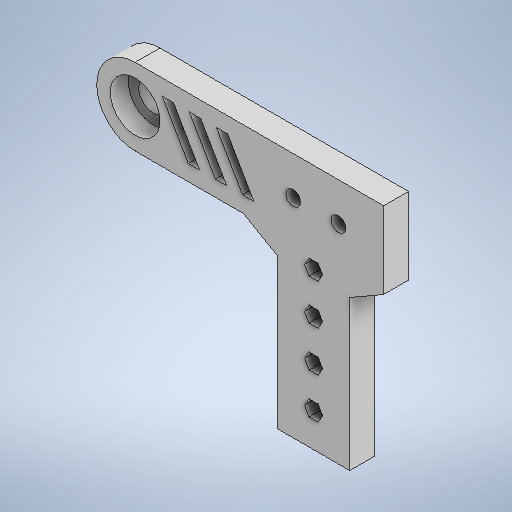
# Autodesk Inventor part: blet_leg_30x30 - rozsirene (zdcardlove)
Saved by Autodesk Inventor 2025 (Build 290162000, 162)
## iProperties
Created: 2024-12-16
Part Number: blet_leg_30x30 - rozsirene (zdcardlove)
Material: Všeobecné
Document SubType Name: Modeling
Designer: lukas
Density: 1 g/cm^3
Appearance: Výchozí
Author: lukas
## iProperties of the stored document blet_leg_30x30_3D tisk.ipt
Created: 2025-01-12
Part Number: blet_leg_30x30_3D tisk
Material: Všeobecné
Document SubType Name: Modeling
Designer: lukas
Density: 1 g/cm^3
Appearance: Výchozí
Author: lukas
Autodesk Inventor part; units mm, degrees
ref_plane "YZ Plane" through (0, 0, 0) normal (1, 0, 0) x (0, 1, 0)
ref_plane "XZ Plane" through (0, 0, 0) normal (0, 1, 0) x (-1, 0, 0)
ref_plane "XY Plane" through (0, 0, 0) normal (0, 0, 1) x (1, 0, 0)
sketch "Náčrt1" plane through (0, 0, 0) normal (0, 0, 1) x (1, 0, 0)
  line L0 (-97.4, 0) -> (80.4, 0) projected
  line L1 (0, -76.3) -> (0, 76.3) projected
  line L2 (-55, 54.5) -> (55, 54.5)
  line L3 (55, 54.5) -> (55, 20.5)
  line L4 (55, 20.5) -> (-55, 20.5)
  line L5 (-55, 20.5) -> (-55, 54.5)
  line L6 (40, -54.5) -> (8, -54.5)
  line L7 (8, -54.5) -> (8, 20.5)
  line L8 (8, 20.5) -> (40, 20.5)
  line L9 (40, 20.5) -> (40, -54.5)
  circle A0 centre (-55, 37.5) radius 17
  point P0 (0, 0)
  point P1 (-55, 20.5)
  dimension "d0" = 34
  dimension "d1" = 110
  dimension "d2" = 32
  dimension "d3" = 15
  dimension "d4" = 75
  constraints: 16 end point, 4 parallel, 2 horizontal, 2 perpendicular, 1 midpoint, 1 point on line, 5 other
  measures "d0" distance of L4.end L2.start
  measures "d1" distance of L2.start L2.end
  measures "d2" distance of L6.start L6.end
  measures "d3" distance from line of L3.end L9
  measures "d4" distance of L6.end L7.end
extrude "Vysunutí1" add sketch "Náčrt1" along normal blind 14 contours L7 L4 L9 L0 | L0 L9 L6 L7 | L4 A0 L2 L1 | L1 L2 L3 L4 | A0 L5 | L5 A0
sketch "Náčrt2" plane through (0, 0, 0) normal (0, 0, -1) x (-1, 0, 0)
  line L0 (-55, 54.5) -> (55, 54.5) projected
  line L1 (-55, 54.5) -> (55, 54.5) projected
  line L2 (-55, 20.5) -> (-55, 54.5) projected
  line L3 (-40, 20.5) -> (-55, 20.5) projected
  line L4 (-40, -54.5) -> (-40, 20.5) projected
  line L5 (-8, -54.5) -> (-40, -54.5) projected
  line L6 (-8, 20.5) -> (-8, -54.5) projected
  line L7 (55, 20.5) -> (-8, 20.5) projected
  arc A0 (55, 20.5) -> (55, 54.5) centre (55, 37.5) ccw projected
  point P0 (0, 0)
  constraints: 1 coincident
hole "Díra1" at (-55, 37.5, 0) direction (0, 0, 1) diameter 13 end through all counterbore diameter 22 counterbore depth 8
chamfer "Zkosení1" distance 3 angle 45 8 edges at (0, 54.5, 14) (-72, 37.5, 14) (-23.5, 20.5, 14) (8, -17, 14) (40, -17, 14) (47.5, 20.5, 14) (55, 37.5, 14) (24, -54.5, 14)
sketch "Náčrt3" plane through (0, 0, 14) normal (0, 0, 1) x (1, 0, 0)
  circle A0 centre (-55, 37.5) radius 6.5 projected
  line L0 (-55, 51.5) -> (52, 51.5) projected
  arc A1 (-55, 51.5) -> (-55, 23.5) centre (-55, 37.5) ccw projected
  line L1 (11, 23.5) -> (-55, 23.5) projected
  line L2 (11, -51.5) -> (11, 23.5) projected
  line L3 (37, -51.5) -> (11, -51.5) projected
  line L4 (37, 23.5) -> (37, -51.5) projected
  line L5 (52, 23.5) -> (37, 23.5) projected
  line L6 (52, 51.5) -> (52, 23.5) projected
  line L7 (0, 76.3) -> (0, -76.3) projected
  line L8 (-97.4, 0) -> (80.4, 0) projected
  point P0 (0, 0)
  point P1 (35, 37.5)
  dimension "d17" = 14
  dimension "d18" = 17
  measures "d17" distance from line of L0 point (35, 37.5)
  measures "d18" distance from line of L6 point (35, 37.5)
hole "Díra2" at (35, 37.5, 14) direction (0, 0, -1) diameter 6.5 end through all counterbore diameter 11 counterbore depth 4 clearance for "Strojní šroub se zápustnou hlavou" size "M6" standard "Ansi M metrický profil"
pattern_linear "Obdélníkové pole1" count 2 spacing 20 along (-1, 0, 0) of "Díra2"
sketch "Náčrt4" plane through (0, 0, 14) normal (0, 0, 1) x (1, 0, 0)
  line L0 (-97.4, 0) -> (80.4, 0) projected
  line L1 (0, -76.3) -> (0, 76.3) projected
  circle A0 centre (15, 37.5) radius 5.5 projected
  circle A1 centre (35, 37.5) radius 5.5 projected
  circle A2 centre (-55, 37.5) radius 6.5 projected
  line L2 (-55, 51.5) -> (52, 51.5) projected
  arc A3 (-55, 51.5) -> (-55, 23.5) centre (-55, 37.5) ccw projected
  line L3 (11, 23.5) -> (-55, 23.5) projected
  line L4 (11, -51.5) -> (11, 23.5) projected
  line L5 (37, -51.5) -> (11, -51.5) projected
  line L6 (37, 23.5) -> (37, -51.5) projected
  line L7 (52, 23.5) -> (37, 23.5) projected
  line L8 (52, 51.5) -> (52, 23.5) projected
  line L9 (-31.453, 27.5) -> (-26.453, 27.5)
  line L10 (-26.453, 27.5) -> (-38, 47.5)
  line L11 (-26.453, 27.5) -> (-3.359, 27.5) construction
  line L12 (-31.453, 27.5) -> (-43, 47.5)
  line L13 (-43, 47.5) -> (-38, 47.5)
  point P0 (0, 0)
  dimension "d29" = 120
  dimension "d31" = 5
  dimension "d32" = 4
  dimension "d33" = 4
  dimension "d34" = 12
  constraints: 10 end point, 3 horizontal, 1 equal length, 1 parallel
  measures "d29" angle of L11 L10
  measures "d31" distance of L12.end L10.end
  measures "d32" distance between parallel lines of L2 L13
  measures "d33" distance between parallel lines of L3 L9
  measures "d34" horizontal distance of A2.centre L12.end
extrude "Vysunutí2" cut sketch "Náčrt4" against normal through all contours L12 L13 L10 L9
chamfer "Zkosení2" distance 1 angle 45 4 edges at (-37.2265, 37.5, 14) (-40.5, 47.5, 14) (-32.2265, 37.5, 14) (-28.953, 27.5, 14)
pattern_linear "Obdélníkové pole2" count 3 spacing 12 along (1, 0, 0) of "Vysunutí2", "Zkosení2"
sketch "Náčrt5" plane through (0, 0, 14) normal (0, 0, 1) x (1, 0, 0)
  line L0 (-32.7321, 48.5) -> (-20.0303, 26.5) projected
  line L1 (-25.4226, 48.5) -> (-32.7321, 48.5) projected
  line L2 (-12.7209, 26.5) -> (-25.4226, 48.5) projected
  line L3 (-20.0303, 26.5) -> (-12.7209, 26.5) projected
  line L4 (-55, 51.5) -> (52, 51.5) projected
  arc A0 (-55, 51.5) -> (-55, 23.5) centre (-55, 37.5) ccw projected
  line L5 (11, 23.5) -> (-55, 23.5) projected
  line L6 (11, -51.5) -> (11, 23.5) projected
  line L7 (37, -51.5) -> (11, -51.5) projected
  line L8 (37, 23.5) -> (37, -51.5) projected
  line L9 (52, 23.5) -> (37, 23.5) projected
  line L10 (52, 51.5) -> (52, 23.5) projected
  circle A1 centre (-55, 37.5) radius 6.5 projected
  circle A2 centre (35, 37.5) radius 5.5 projected
  circle A3 centre (15, 37.5) radius 5.5 projected
  line L11 (-24.7209, 26.5) -> (-37.4226, 48.5) projected
  line L12 (-32.0303, 26.5) -> (-24.7209, 26.5) projected
  line L13 (-44.7321, 48.5) -> (-32.0303, 26.5) projected
  line L14 (-37.4226, 48.5) -> (-44.7321, 48.5) projected
  line L15 (-20.7321, 48.5) -> (-8.0303, 26.5) projected
  line L16 (-13.4226, 48.5) -> (-20.7321, 48.5) projected
  line L17 (-0.7209, 26.5) -> (-13.4226, 48.5) projected
  line L18 (-8.0303, 26.5) -> (-0.7209, 26.5) projected
  line L19 (0, -76.3) -> (0, 76.3) projected
  line L20 (26, 17.9641) -> (28, 14.5)
  line L21 (28, 14.5) -> (26, 11.0359)
  line L22 (26, 11.0359) -> (22, 11.0359)
  line L23 (22, 11.0359) -> (20, 14.5)
  line L24 (20, 14.5) -> (22, 17.9641)
  line L25 (22, 17.9641) -> (26, 17.9641)
  point P0 (0, 0)
  point P1 (24, 14.5)
  dimension "d43" = 4
  dimension "d44" = 9
  dimension "d45" = 13
  dimension "d52" = 3.4641
  constraints: 12 end point, 13 other
  measures "d43" distance of L24.end L20.start
  measures "d44" distance from line of L9 point (24, 14.5)
  measures "d45" distance from line of L8 point (24, 14.5)
  measures "d52" vertical distance of L23.end L24.end
extrude "Vysunutí3" cut sketch "Náčrt5" against normal through all contours L20 L21 L22 L23 L24 L25
chamfer "Zkosení3" distance 1 angle 45 6 edges at (24, 17.9641, 14) (27, 16.2321, 14) (27, 12.7679, 14) (24, 11.0359, 14) (21, 12.7679, 14) (21, 16.2321, 14)
pattern_linear "Obdélníkové pole3" count 4 spacing 18 along (0, -1, 0) of "Vysunutí3", "Zkosení3"
ref_plane "Pracovní rovina1" through (0, 0, 0) normal (0, 0, -1) x (-1, 0, 0)
sketch "Náčrt7" plane through (0, 0, 0) normal (0, 0, -1) x (-1, 0, 0)
  line L0 (-28, -39.5) -> (-26, -36.0359) projected
  line L1 (-26, -36.0359) -> (-22, -36.0359) projected
  line L2 (-22, -36.0359) -> (-20, -39.5) projected
  line L3 (-20, -39.5) -> (-22, -42.9641) projected
  line L4 (-22, -42.9641) -> (-26, -42.9641) projected
  line L5 (-26, -42.9641) -> (-28, -39.5) projected
  line L6 (-28, -21.5) -> (-26, -18.0359) projected
  line L7 (-26, -18.0359) -> (-22, -18.0359) projected
  line L8 (-22, -18.0359) -> (-20, -21.5) projected
  line L9 (-20, -21.5) -> (-22, -24.9641) projected
  line L10 (-22, -24.9641) -> (-26, -24.9641) projected
  line L11 (-26, -24.9641) -> (-28, -21.5) projected
  line L12 (-28, -3.5) -> (-26, -0.0359) projected
  line L13 (-26, -0.0359) -> (-22, -0.0359) projected
  line L14 (-22, -0.0359) -> (-20, -3.5) projected
  line L15 (-20, -3.5) -> (-22, -6.9641) projected
  line L16 (-22, -6.9641) -> (-26, -6.9641) projected
  line L17 (-26, -6.9641) -> (-28, -3.5) projected
  line L18 (-20, 14.5) -> (-22, 11.0359) projected
  line L19 (-22, 11.0359) -> (-26, 11.0359) projected
  line L20 (-26, 11.0359) -> (-28, 14.5) projected
  line L21 (-28, 14.5) -> (-26, 17.9641) projected
  line L22 (-26, 17.9641) -> (-22, 17.9641) projected
  line L23 (-22, 17.9641) -> (-20, 14.5) projected
  line L24 (19, 47.5) -> (7.453, 27.5) projected
  line L25 (7.453, 27.5) -> (2.453, 27.5) projected
  line L26 (2.453, 27.5) -> (14, 47.5) projected
  line L27 (14, 47.5) -> (19, 47.5) projected
  line L28 (31, 47.5) -> (19.453, 27.5) projected
  line L29 (19.453, 27.5) -> (14.453, 27.5) projected
  line L30 (14.453, 27.5) -> (26, 47.5) projected
  line L31 (26, 47.5) -> (31, 47.5) projected
  line L32 (26.453, 27.5) -> (38, 47.5) projected
  line L33 (38, 47.5) -> (43, 47.5) projected
  line L34 (43, 47.5) -> (31.453, 27.5) projected
  line L35 (31.453, 27.5) -> (26.453, 27.5) projected
  circle A0 centre (-15, 37.5) radius 3.25 projected
  circle A1 centre (-35, 37.5) radius 3.25 projected
  circle A2 centre (55, 37.5) radius 11 projected
  line L36 (-55, 54.5) -> (55, 54.5) projected
  line L37 (-55, 20.5) -> (-55, 54.5) projected
  line L38 (-40, 20.5) -> (-55, 20.5) projected
  line L39 (-40, -54.5) -> (-40, 20.5) projected
  line L40 (-8, -54.5) -> (-40, -54.5) projected
  line L41 (-8, 20.5) -> (-8, -54.5) projected
  line L42 (55, 20.5) -> (-8, 20.5) projected
  arc A3 (55, 20.5) -> (55, 54.5) centre (55, 37.5) ccw projected
  line L43 (-40, 11.8397) -> (-55, 20.5)
  line L44 (-8, 11.8397) -> (7, 20.5)
  line L45 (-8, 20.5) -> (-8, -54.5) projected
  line L46 (-8, 11.8397) -> (-8, 20.5)
  line L47 (-8, 20.5) -> (7, 20.5)
  line L48 (-40, -54.5) -> (-40, 20.5) projected
  line L49 (-40, 11.8397) -> (-40, 20.5)
  line L50 (-40, 20.5) -> (-55, 20.5)
  point P0 (0, 0)
  dimension "d68" = 15
  dimension "d69" = 15
  dimension "d70" = 30
  dimension "d71" = 30
  constraints: 12 end point, 4 collinear, 4 point on line
  measures "d68" distance of L38.start L43.end
  measures "d69" distance of L41.start L44.end
  measures "d70" angle of L42 L44
  measures "d71" angle of L38 L43
extrude "Vysunutí4" add sketch "Náčrt7" against normal blind 11 contours L38 L39 L43 | L44 L41 L42
mirror "Zrcadlit1" about plane through (0, 0, 0) normal (0, 0, 1) remove original yes
